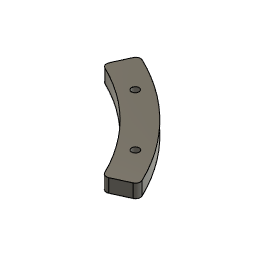
JL Audio_13TW5v2_Subwoofer_Bracket_ v1 (Autodesk Fusion 360 design; units mm, degrees)
Autodesk Fusion 360 part; units mm, degrees
sketch "Sketch1" plane through (0, 0, 0) normal (0, 1, 0) x (1, 0, 0)
  circle A0 centre (0, 0) radius 183
  circle A1 centre (0, 0) radius 160
  circle A2 centre (0, 0) radius 171.5 construction
  dimension "d1" = 366
  dimension "d2" = 320
  dimension "d3" = 343
  constraint coincident A0.centre A1.centre
  constraint concentric A1 A2
  measures "d1" diameter of A0
  measures "d2" diameter of A1
  measures "d3" diameter of A2
sketch "Sketch2" plane through (0, 0, 0) normal (0, 1, 0) x (1, 0, 0)
  circle A0 centre (97.8605, 140.8388) radius 3.06
  circle A1 centre (0, 0) radius 171.5
  circle A2 centre (140.5474, 98.2785) radius 3.06
  dimension "d4" = 6.12
  dimension "d5" = 6.12
  constraint coincident A0.centre A1
  constraint coincident A1 A2.centre
  measures "d4" diameter of A0
  measures "d5" diameter of A2
sketch "Sketch3" plane through (0, 0, 0) normal (0, 1, 0) x (1, 0, 0)
  circle A0 centre (0, 0) radius 183
  line L0 (0, 0) -> (75.9151, 166.511)
  line L1 (0, 0) -> (166.6348, 75.6428)
  constraint coincident A0.centre L0.start
  constraint coincident A0 L0.end
  constraint coincident A0 L1.end
extrude "Extrude2" add sketch "Sketch3" against normal blind 11 contours A0 L0 L1 picked at (86.1157, 85.9751)
extrude "Extrude3" cut sketch "Sketch1" against normal up to surface (11 mm away) contours A1
extrude "Extrude4" cut sketch "Sketch2" against normal up to surface (11 mm away) contours A0 A1 | A0 A1 | A1 A2 | A1 A2
fillet "Fillet1" radius 4 4 edges at (166.6348, -5.5, -75.6428) (145.6916, -5.5, -66.1358) (66.3738, -5.5, -145.5834) (75.9151, -5.5, -166.511)
